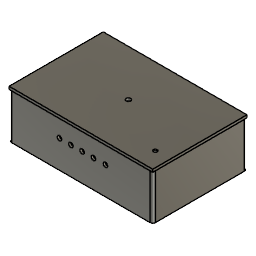
Modelado 3D rehechov2 (Autodesk Fusion 360 design; units mm, degrees)
part number: 2026-04-29-23-24-20-997
part number: 2026-04-29-23-24-29-026
Autodesk Fusion 360 part; units mm, degrees
sketch "Boceto1" plane through (0, 0, 0) normal (0, 0, 1) x (1, 0, 0) in component "PrototipoUV_CajaReal"
  line L0 (0, 0) -> (160, 0)
  line L1 (160, 0) -> (160, 105)
  line L2 (160, 105) -> (0, 105)
  line L3 (0, 105) -> (0, 0)
extrude "Extruir1" add sketch "Boceto1" along normal blind 50 makes body 1 in component "PrototipoUV_CajaReal"
fillet "Empalme1" radius 3 4 edges at (0, 105, 25) (160, 105, 25) (160, 0, 25) (0, 0, 25) on bodies 1 in component "PrototipoUV_CajaReal"
shell "Vaciado1" thickness 2.5 removed faces 1 at (105.6667, 35, 50) on bodies 1 in component "PrototipoUV_CajaReal"
ref_plane "PlanoDeObra1" through (0, 0, 50) normal (0, 0, 1) x (1, 0, 0) in component "PrototipoUV_CajaReal"
sketch "Boceto2" plane through (0, 0, 50) normal (0, 0, 1) x (1, 0, 0) in component "PrototipoUV_CajaReal"
  line L0 (0, 0) -> (160, 0)
  line L1 (160, 0) -> (160, 105)
  line L2 (160, 105) -> (0, 105)
  line L3 (0, 105) -> (0, 0)
extrude "Extruir2" add sketch "Boceto2" along normal blind 3 separate body makes body 2 in component "PrototipoUV_CajaReal"
ref_plane "PlanoDeObra2" through (0, 0, 46.5) normal (0, 0, 1) x (1, 0, 0) in component "PrototipoUV_CajaReal"
sketch "Boceto3" plane through (0, 0, 46.5) normal (0, 0, 1) x (1, 0, 0) in component "PrototipoUV_CajaReal"
  line L0 (3.7, 3.7) -> (156.3, 3.7)
  line L1 (156.3, 3.7) -> (156.3, 101.3)
  line L2 (156.3, 101.3) -> (3.7, 101.3)
  line L3 (3.7, 101.3) -> (3.7, 3.7)
extrude "Extruir3" add sketch "Boceto3" along normal blind 3.5 separate body makes body 3 in component "PrototipoUV_CajaReal"
ref_plane "PlanoDeObra3" through (0, 0, 53.3) normal (0, 0, 1) x (1, 0, 0) in component "PrototipoUV_CajaReal"
sketch "Boceto4" plane through (0, 0, 53.3) normal (0, 0, 1) x (1, 0, 0) in component "PrototipoUV_CajaReal"
  line L0 (30, 12.5) -> (130, 12.5)
  line L1 (130, 12.5) -> (130, 92.5)
  line L2 (130, 92.5) -> (30, 92.5)
  line L3 (30, 92.5) -> (30, 12.5)
ref_plane "PlanoDeObra4" through (0, 0, 55.2) normal (0, 0, 1) x (1, 0, 0) in component "PrototipoUV_CajaReal"
sketch "Boceto5" plane through (0, 0, 55.2) normal (0, 0, 1) x (1, 0, 0) in component "PrototipoUV_CajaReal"
  line L0 (30, 12.5) -> (130, 12.5)
  line L1 (130, 12.5) -> (130, 13.7)
  line L2 (130, 13.7) -> (30, 13.7)
  line L3 (30, 13.7) -> (30, 12.5)
ref_plane "PlanoDeObra5" through (0, 0, 55.2) normal (0, 0, 1) x (1, 0, 0) in component "PrototipoUV_CajaReal"
sketch "Boceto6" plane through (0, 0, 55.2) normal (0, 0, 1) x (1, 0, 0) in component "PrototipoUV_CajaReal"
  line L0 (30, 91.3) -> (130, 91.3)
  line L1 (130, 91.3) -> (130, 92.5)
  line L2 (130, 92.5) -> (30, 92.5)
  line L3 (30, 92.5) -> (30, 91.3)
ref_plane "PlanoDeObra6" through (0, 0, 55.2) normal (0, 0, 1) x (1, 0, 0) in component "PrototipoUV_CajaReal"
sketch "Boceto7" plane through (0, 0, 55.2) normal (0, 0, 1) x (1, 0, 0) in component "PrototipoUV_CajaReal"
  line L0 (30, 12.5) -> (31.2, 12.5)
  line L1 (31.2, 12.5) -> (31.2, 92.5)
  line L2 (31.2, 92.5) -> (30, 92.5)
  line L3 (30, 92.5) -> (30, 12.5)
ref_plane "PlanoDeObra7" through (0, 0, 55.2) normal (0, 0, 1) x (1, 0, 0) in component "PrototipoUV_CajaReal"
sketch "Boceto8" plane through (0, 0, 55.2) normal (0, 0, 1) x (1, 0, 0) in component "PrototipoUV_CajaReal"
  line L0 (128.8, 12.5) -> (130, 12.5)
  line L1 (130, 12.5) -> (130, 92.5)
  line L2 (130, 92.5) -> (128.8, 92.5)
  line L3 (128.8, 92.5) -> (128.8, 12.5)
ref_plane "PlanoDeObra8" through (0, 0, 55.25) normal (0, 0, 1) x (1, 0, 0) in component "PrototipoUV_CajaReal"
sketch "Boceto9" plane through (0, 0, 55.25) normal (0, 0, 1) x (1, 0, 0) in component "PrototipoUV_CajaReal"
  line L0 (54.75, 14) -> (55.25, 14)
  line L1 (55.25, 14) -> (55.25, 91)
  line L2 (55.25, 91) -> (54.75, 91)
  line L3 (54.75, 91) -> (54.75, 14)
ref_plane "PlanoDeObra9" through (0, 0, 55.25) normal (0, 0, 1) x (1, 0, 0) in component "PrototipoUV_CajaReal"
sketch "Boceto10" plane through (0, 0, 55.25) normal (0, 0, 1) x (1, 0, 0) in component "PrototipoUV_CajaReal"
  line L0 (79.75, 14) -> (80.25, 14)
  line L1 (80.25, 14) -> (80.25, 91)
  line L2 (80.25, 91) -> (79.75, 91)
  line L3 (79.75, 91) -> (79.75, 14)
ref_plane "PlanoDeObra10" through (0, 0, 55.25) normal (0, 0, 1) x (1, 0, 0) in component "PrototipoUV_CajaReal"
sketch "Boceto11" plane through (0, 0, 55.25) normal (0, 0, 1) x (1, 0, 0) in component "PrototipoUV_CajaReal"
  line L0 (104.75, 14) -> (105.25, 14)
  line L1 (105.25, 14) -> (105.25, 91)
  line L2 (105.25, 91) -> (104.75, 91)
  line L3 (104.75, 91) -> (104.75, 14)
ref_plane "PlanoDeObra11" through (0, 0, 55.25) normal (0, 0, 1) x (1, 0, 0) in component "PrototipoUV_CajaReal"
sketch "Boceto12" plane through (0, 0, 55.25) normal (0, 0, 1) x (1, 0, 0) in component "PrototipoUV_CajaReal"
  line L0 (31.5, 38.9167) -> (128.5, 38.9167)
  line L1 (128.5, 38.9167) -> (128.5, 39.4167)
  line L2 (128.5, 39.4167) -> (31.5, 39.4167)
  line L3 (31.5, 39.4167) -> (31.5, 38.9167)
ref_plane "PlanoDeObra12" through (0, 0, 55.25) normal (0, 0, 1) x (1, 0, 0) in component "PrototipoUV_CajaReal"
sketch "Boceto13" plane through (0, 0, 55.25) normal (0, 0, 1) x (1, 0, 0) in component "PrototipoUV_CajaReal"
  line L0 (31.5, 65.5833) -> (128.5, 65.5833)
  line L1 (128.5, 65.5833) -> (128.5, 66.0833)
  line L2 (128.5, 66.0833) -> (31.5, 66.0833)
  line L3 (31.5, 66.0833) -> (31.5, 65.5833)
ref_plane "PlanoDeObra13" through (0, 0, 53.3) normal (0, 0, 1) x (1, 0, 0) in component "PrototipoUV_CajaReal"
sketch "Boceto14" plane through (0, 0, 53.3) normal (0, 0, 1) x (1, 0, 0) in component "PrototipoUV_CajaReal"
  line L0 (134.5, 17.5) -> (151.5, 17.5)
  line L1 (151.5, 17.5) -> (151.5, 32.5)
  line L2 (151.5, 32.5) -> (134.5, 32.5)
  line L3 (134.5, 32.5) -> (134.5, 17.5)
ref_plane "PlanoDeObra14" through (0, 0, 54.6) normal (0, 0, 1) x (1, 0, 0) in component "PrototipoUV_CajaReal"
sketch "Boceto15" plane through (0, 0, 54.6) normal (0, 0, 1) x (1, 0, 0) in component "PrototipoUV_CajaReal"
  circle A0 centre (143, 25) radius 2.8
ref_plane "PlanoDeObra15" through (0, -0.6, 0) normal (0, 1, 0) x (0, 0, 1) in component "PrototipoUV_CajaReal"
sketch "Boceto16" plane through (0, -0.6, 0) normal (0, 1, 0) x (1, 0, 0) in component "PrototipoUV_CajaReal"
  circle A0 centre (80, 23.5) radius 4
ref_plane "PlanoDeObra16" through (0, 105.1, 0) normal (0, 1, 0) x (0, 0, 1) in component "PrototipoUV_CajaReal"
sketch "Boceto17" plane through (0, 105.1, 0) normal (0, 1, 0) x (1, 0, 0) in component "PrototipoUV_CajaReal"
  circle A0 centre (108, 16) radius 1.25
ref_plane "PlanoDeObra17" through (0, 105.1, 0) normal (0, 1, 0) x (0, 0, 1) in component "PrototipoUV_CajaReal"
sketch "Boceto18" plane through (0, 105.1, 0) normal (0, 1, 0) x (1, 0, 0) in component "PrototipoUV_CajaReal"
  circle A0 centre (113.5, 16) radius 1.25
ref_plane "PlanoDeObra18" through (0, 105.1, 0) normal (0, 1, 0) x (0, 0, 1) in component "PrototipoUV_CajaReal"
sketch "Boceto19" plane through (0, 105.1, 0) normal (0, 1, 0) x (1, 0, 0) in component "PrototipoUV_CajaReal"
  circle A0 centre (119, 16) radius 1.25
ref_plane "PlanoDeObra19" through (0, 105.1, 0) normal (0, 1, 0) x (0, 0, 1) in component "PrototipoUV_CajaReal"
sketch "Boceto20" plane through (0, 105.1, 0) normal (0, 1, 0) x (1, 0, 0) in component "PrototipoUV_CajaReal"
  circle A0 centre (124.5, 16) radius 1.25
ref_plane "PlanoDeObra20" through (0, 105.1, 0) normal (0, 1, 0) x (0, 0, 1) in component "PrototipoUV_CajaReal"
sketch "Boceto21" plane through (0, 105.1, 0) normal (0, 1, 0) x (1, 0, 0) in component "PrototipoUV_CajaReal"
  circle A0 centre (130, 16) radius 1.25
ref_plane "PlanoDeObra21" through (0, 105.1, 0) normal (0, 1, 0) x (0, 0, 1) in component "PrototipoUV_CajaReal"
sketch "Boceto22" plane through (0, 105.1, 0) normal (0, 1, 0) x (1, 0, 0) in component "PrototipoUV_CajaReal"
  circle A0 centre (135.5, 16) radius 1.25
ref_plane "PlanoDeObra22" through (0, 105.1, 0) normal (0, 1, 0) x (0, 0, 1) in component "PrototipoUV_CajaReal"
sketch "Boceto23" plane through (0, 105.1, 0) normal (0, 1, 0) x (1, 0, 0) in component "PrototipoUV_CajaReal"
  circle A0 centre (141, 16) radius 1.25
ref_plane "PlanoDeObra23" through (0, 105.1, 0) normal (0, 1, 0) x (0, 0, 1) in component "PrototipoUV_CajaReal"
sketch "Boceto24" plane through (0, 105.1, 0) normal (0, 1, 0) x (1, 0, 0) in component "PrototipoUV_CajaReal"
  circle A0 centre (146.5, 16) radius 1.25
ref_plane "PlanoDeObra24" through (0, 105.1, 0) normal (0, 1, 0) x (0, 0, 1) in component "PrototipoUV_CajaReal"
sketch "Boceto25" plane through (0, 105.1, 0) normal (0, 1, 0) x (1, 0, 0) in component "PrototipoUV_CajaReal"
  circle A0 centre (108, 21.5) radius 1.25
ref_plane "PlanoDeObra25" through (0, 105.1, 0) normal (0, 1, 0) x (0, 0, 1) in component "PrototipoUV_CajaReal"
sketch "Boceto26" plane through (0, 105.1, 0) normal (0, 1, 0) x (1, 0, 0) in component "PrototipoUV_CajaReal"
  circle A0 centre (113.5, 21.5) radius 1.25
ref_plane "PlanoDeObra26" through (0, 105.1, 0) normal (0, 1, 0) x (0, 0, 1) in component "PrototipoUV_CajaReal"
sketch "Boceto27" plane through (0, 105.1, 0) normal (0, 1, 0) x (1, 0, 0) in component "PrototipoUV_CajaReal"
  circle A0 centre (119, 21.5) radius 1.25
ref_plane "PlanoDeObra27" through (0, 105.1, 0) normal (0, 1, 0) x (0, 0, 1) in component "PrototipoUV_CajaReal"
sketch "Boceto28" plane through (0, 105.1, 0) normal (0, 1, 0) x (1, 0, 0) in component "PrototipoUV_CajaReal"
  circle A0 centre (124.5, 21.5) radius 1.25
ref_plane "PlanoDeObra28" through (0, 105.1, 0) normal (0, 1, 0) x (0, 0, 1) in component "PrototipoUV_CajaReal"
sketch "Boceto29" plane through (0, 105.1, 0) normal (0, 1, 0) x (1, 0, 0) in component "PrototipoUV_CajaReal"
  circle A0 centre (130, 21.5) radius 1.25
ref_plane "PlanoDeObra29" through (0, 105.1, 0) normal (0, 1, 0) x (0, 0, 1) in component "PrototipoUV_CajaReal"
sketch "Boceto30" plane through (0, 105.1, 0) normal (0, 1, 0) x (1, 0, 0) in component "PrototipoUV_CajaReal"
  circle A0 centre (135.5, 21.5) radius 1.25
ref_plane "PlanoDeObra30" through (0, 105.1, 0) normal (0, 1, 0) x (0, 0, 1) in component "PrototipoUV_CajaReal"
sketch "Boceto31" plane through (0, 105.1, 0) normal (0, 1, 0) x (1, 0, 0) in component "PrototipoUV_CajaReal"
  circle A0 centre (141, 21.5) radius 1.25
ref_plane "PlanoDeObra31" through (0, 105.1, 0) normal (0, 1, 0) x (0, 0, 1) in component "PrototipoUV_CajaReal"
sketch "Boceto32" plane through (0, 105.1, 0) normal (0, 1, 0) x (1, 0, 0) in component "PrototipoUV_CajaReal"
  circle A0 centre (146.5, 21.5) radius 1.25
ref_plane "PlanoDeObra32" through (0, 105.1, 0) normal (0, 1, 0) x (0, 0, 1) in component "PrototipoUV_CajaReal"
sketch "Boceto33" plane through (0, 105.1, 0) normal (0, 1, 0) x (1, 0, 0) in component "PrototipoUV_CajaReal"
  circle A0 centre (108, 27) radius 1.25
ref_plane "PlanoDeObra33" through (0, 105.1, 0) normal (0, 1, 0) x (0, 0, 1) in component "PrototipoUV_CajaReal"
sketch "Boceto34" plane through (0, 105.1, 0) normal (0, 1, 0) x (1, 0, 0) in component "PrototipoUV_CajaReal"
  circle A0 centre (113.5, 27) radius 1.25
ref_plane "PlanoDeObra34" through (0, 105.1, 0) normal (0, 1, 0) x (0, 0, 1) in component "PrototipoUV_CajaReal"
sketch "Boceto35" plane through (0, 105.1, 0) normal (0, 1, 0) x (1, 0, 0) in component "PrototipoUV_CajaReal"
  circle A0 centre (119, 27) radius 1.25
ref_plane "PlanoDeObra35" through (0, 105.1, 0) normal (0, 1, 0) x (0, 0, 1) in component "PrototipoUV_CajaReal"
sketch "Boceto36" plane through (0, 105.1, 0) normal (0, 1, 0) x (1, 0, 0) in component "PrototipoUV_CajaReal"
  circle A0 centre (124.5, 27) radius 1.25
ref_plane "PlanoDeObra36" through (0, 105.1, 0) normal (0, 1, 0) x (0, 0, 1) in component "PrototipoUV_CajaReal"
sketch "Boceto37" plane through (0, 105.1, 0) normal (0, 1, 0) x (1, 0, 0) in component "PrototipoUV_CajaReal"
  circle A0 centre (130, 27) radius 1.25
ref_plane "PlanoDeObra37" through (0, 105.1, 0) normal (0, 1, 0) x (0, 0, 1) in component "PrototipoUV_CajaReal"
sketch "Boceto38" plane through (0, 105.1, 0) normal (0, 1, 0) x (1, 0, 0) in component "PrototipoUV_CajaReal"
  circle A0 centre (135.5, 27) radius 1.25
ref_plane "PlanoDeObra38" through (0, 105.1, 0) normal (0, 1, 0) x (0, 0, 1) in component "PrototipoUV_CajaReal"
sketch "Boceto39" plane through (0, 105.1, 0) normal (0, 1, 0) x (1, 0, 0) in component "PrototipoUV_CajaReal"
  circle A0 centre (141, 27) radius 1.25
ref_plane "PlanoDeObra39" through (0, 105.1, 0) normal (0, 1, 0) x (0, 0, 1) in component "PrototipoUV_CajaReal"
sketch "Boceto40" plane through (0, 105.1, 0) normal (0, 1, 0) x (1, 0, 0) in component "PrototipoUV_CajaReal"
  circle A0 centre (146.5, 27) radius 1.25
ref_plane "PlanoDeObra40" through (0, 0, 3) normal (0, 0, 1) x (1, 0, 0) in component "PrototipoUV_CajaReal"
sketch "Boceto41" plane through (0, 0, 3) normal (0, 0, 1) x (1, 0, 0) in component "PrototipoUV_CajaReal"
  line L0 (12.5, 12.5) -> (75.5, 12.5)
  line L1 (75.5, 12.5) -> (75.5, 39.5)
  line L2 (75.5, 39.5) -> (12.5, 39.5)
  line L3 (12.5, 39.5) -> (12.5, 12.5)
ref_plane "PlanoDeObra41" through (0, 0, 3) normal (0, 0, 1) x (1, 0, 0) in component "PrototipoUV_CajaReal"
sketch "Boceto42" plane through (0, 0, 3) normal (0, 0, 1) x (1, 0, 0) in component "PrototipoUV_CajaReal"
  line L0 (94, 12.5) -> (149, 12.5)
  line L1 (149, 12.5) -> (149, 47.5)
  line L2 (149, 47.5) -> (94, 47.5)
  line L3 (94, 47.5) -> (94, 12.5)
sketch "Boceto1 (2)" plane through (0, 0, 0) normal (0, -1, 0) x (1, 0, 0)
  line L0 (3, 50) -> (3, 0)
  line L1 (3, 0) -> (157, 0)
  line L2 (157, 0) -> (157, 50)
  line L3 (157, 50) -> (3, 50)
hole "Agujero1" at (80, 105, 25) direction (0, -1, 0) diameter 8 depth 5 tip angle 118 bodies 1 in component "PrototipoUV_CajaReal"
sketch "Boceto2 (2)" plane through (0, 0, 0) normal (0, 1, 0) x (1, 0, 0)
sketch "Boceto3 (2)" plane through (0, 0, 0) normal (0, 1, 0) x (1, 0, 0)
sketch "Boceto4 (2)" plane through (0, 0, 0) normal (0, 1, 0) x (1, 0, 0)
  circle A0 centre (40, -30) radius 2.5
  circle A1 centre (40, -30) radius 2.5
  circle A2 centre (50, -30) radius 2.5
  circle A3 centre (60, -30) radius 2.5
  circle A4 centre (70, -30) radius 2.5
  circle A5 centre (80, -30) radius 2.5
  circle A6 centre (90, -30) radius 2.5
  circle A7 centre (100, -30) radius 2.5
  dimension "d132" = 5
  dimension "d133" = 5
  dimension "d134" = 5
  dimension "d135" = 5
  dimension "d136" = 5
  dimension "d137" = 5
  dimension "d138" = 5
  dimension "d139" = 5
  measures "d132" diameter of A0
  measures "d133" diameter of A1
  measures "d134" diameter of A2
  measures "d135" diameter of A3
  measures "d136" diameter of A4
  measures "d137" diameter of A5
  measures "d138" diameter of A6
  measures "d139" diameter of A7
hole "Agujero9" at (107.3794, 2.5, 30.9159) direction (0, -1, 0) diameter 5 depth 30 tip angle 118 bodies 1 in component "PrototipoUV_CajaReal"
hole "Agujero10" at (94.084, 2.5, 30.8935) direction (0, -1, 0) diameter 5 depth 30 tip angle 118 bodies 1 in component "PrototipoUV_CajaReal"
hole "Agujero11" at (81.3834, 2.5, 30.8721) direction (0, -1, 0) diameter 5 depth 30 tip angle 118 bodies 1 in component "PrototipoUV_CajaReal"
hole "Agujero12" at (68.9096, 2.5, 30.8512) direction (0, -1, 0) diameter 5 depth 30 tip angle 118 bodies 1 in component "PrototipoUV_CajaReal"
hole "Agujero13" at (56.209, 2.5, 31.0624) direction (0, -1, 0) diameter 5 depth 30 tip angle 118 bodies 1 in component "PrototipoUV_CajaReal"
sketch "Boceto9 (2)" plane through (0, 0, 2.5) normal (0, 0, 1) x (-1, 0, 0)
  arc A0 (-2.5, -3) -> (-3, -2.5) centre (-3, -3) ccw
  line L0 (-3, -2.5) -> (-157, -2.5)
  arc A1 (-157, -2.5) -> (-157.5, -3) centre (-157, -3) ccw
  line L1 (-157.5, -3) -> (-157.5, -102)
  arc A2 (-157.5, -102) -> (-157, -102.5) centre (-157, -102) ccw
  line L2 (-157, -102.5) -> (-3, -102.5)
  arc A3 (-3, -102.5) -> (-2.5, -102) centre (-3, -102) ccw
  line L3 (-2.5, -102) -> (-2.5, -3)
  line L4 (-150, -10) -> (-94, -10)
  line L5 (-94, -10) -> (-94, -13)
  line L6 (-94, -13) -> (-150, -13)
  line L7 (-150, -13) -> (-150, -10)
  line L8 (-147.3696, -10) -> (-150.3696, -10)
  line L9 (-150.3696, -10) -> (-150.3696, -45)
  line L10 (-150.3696, -45) -> (-147.3696, -45)
  line L11 (-147.3696, -45) -> (-147.3696, -10)
  line L12 (-150.3696, -41.6297) -> (-94.3696, -41.6297)
  line L13 (-94.3696, -41.6297) -> (-94.3696, -45)
  line L14 (-94.3696, -45) -> (-150.3696, -45)
  line L15 (-150.3696, -45) -> (-150.3696, -41.6297)
  dimension "d190" = 56
  dimension "d191" = 3
  dimension "d192" = 3
  dimension "d193" = 35
  dimension "d194" = 56
  constraint horizontal L4
  constraint vertical L5
  constraint horizontal L6
  constraint vertical L7
  constraint horizontal L8
  constraint vertical L9
  constraint horizontal L10
  constraint vertical L11
  constraint coincident L4 L8.start
  constraint horizontal L12
  constraint vertical L13
  constraint horizontal L14
  constraint vertical L15
  constraint coincident L9 L12.start
  measures "d190" distance of L4.start L4.end
  measures "d191" distance of L4.start L6.end
  measures "d192" distance of L8.start L8.end
  measures "d193" distance of L8.start L10.end
  measures "d194" distance of L12.start L12.end
extrude "Extruir46" add sketch "Boceto9 (2)" along normal blind 10 contours L4 L6 L7 L8 L11 | L6 L7 L8 L9 L11 L12 | L4 L5 L6 L11 | L9 L10 L11 L12 L14 L15 | L11 L12 L13 L14 bodies 1 in component "PrototipoUV_CajaReal"
sketch "Boceto10 (2)" plane through (0, 0, 4.5) normal (0, 0, 1) x (-1, 0, 0)
  line L0 (-12.5, -39.5) -> (-12.5, -12.5)
  line L1 (-12.5, -12.5) -> (-75.5, -12.5)
  line L2 (-75.5, -12.5) -> (-75.5, -39.5)
  line L3 (-75.5, -39.5) -> (-12.5, -39.5)
  line L4 (-150, -52.9904) -> (-82, -52.9904)
  line L5 (-82, -52.9904) -> (-82, -49.9904)
  line L6 (-82, -49.9904) -> (-150, -49.9904)
  line L7 (-150, -49.9904) -> (-150, -52.9904)
  line L8 (-150, -49.9904) -> (-147, -49.9904)
  line L9 (-147, -49.9904) -> (-147, -100.9904)
  line L10 (-147, -100.9904) -> (-150, -100.9904)
  line L11 (-150, -100.9904) -> (-150, -49.9904)
  line L12 (-150, -100.9904) -> (-82, -100.9904)
  line L13 (-82, -100.9904) -> (-82, -97.9904)
  line L14 (-82, -97.9904) -> (-150, -97.9904)
  line L15 (-150, -97.9904) -> (-150, -100.9904)
  dimension "d197" = 68
  dimension "d198" = 3
  dimension "d199" = 3
  dimension "d200" = 51
  dimension "d201" = 68
  dimension "d202" = 3
  constraint horizontal L4
  constraint vertical L5
  constraint horizontal L6
  constraint vertical L7
  constraint horizontal L8
  constraint vertical L9
  constraint horizontal L10
  constraint vertical L11
  constraint horizontal L12
  constraint vertical L13
  constraint horizontal L14
  constraint vertical L15
  measures "d197" distance of L4.start L4.end
  measures "d198" distance of L4.start L6.end
  measures "d199" distance of L6.end L8.end
  measures "d200" distance of L6.end L10.end
  measures "d201" distance of L10.end L12.end
  measures "d202" distance of L10.end L14.end
extrude "Extruir1'" add sketch "Boceto10 (2)" along normal blind 9 separate body contours L4 L6 L7 L8 L9 L11 | L4 L9 L11 L14 | L4 L5 L6 L9 | L9 L10 L11 L12 L14 L15 | L9 L12 L13 L14 makes body 4
hole "Agujero14" at (143.6047, 19.3786, 53) direction (0, 0, -1) diameter 3.3 depth 7 tip angle 180 countersink diameter 4.4 countersink angle 90 bodies 2 3 in component "PrototipoUV_CajaReal"
hole "Agujero17" at (79.3666, 53.5561, 53) direction (0, 0, -1) diameter 5 depth 7 tip angle 180 bodies 2 3 in component "PrototipoUV_CajaReal"
sketch "Boceto11 (2)" plane through (0, 0, 2.5) normal (0, 0, 1) x (-1, 0, 0)
  line L0 (-147.3696, -41.6297) -> (-94.3696, -41.6297)
  line L1 (-94.3696, -41.6297) -> (-94.3696, -45)
  line L2 (-94.3696, -45) -> (-150.3696, -45)
  line L3 (-150.3696, -45) -> (-150.3696, -10)
  line L4 (-150.3696, -10) -> (-94, -10)
  line L5 (-94, -10) -> (-94, -13)
  line L6 (-94, -13) -> (-147.3696, -13)
  line L7 (-147.3696, -13) -> (-147.3696, -41.6297)
  arc A0 (-2.5, -3) -> (-3, -2.5) centre (-3, -3) ccw
  line L8 (-3, -2.5) -> (-157, -2.5)
  arc A1 (-157, -2.5) -> (-157.5, -3) centre (-157, -3) ccw
  line L9 (-157.5, -3) -> (-157.5, -102)
  arc A2 (-157.5, -102) -> (-157, -102.5) centre (-157, -102) ccw
  line L10 (-157, -102.5) -> (-3, -102.5)
  arc A3 (-3, -102.5) -> (-2.5, -102) centre (-3, -102) ccw
  line L11 (-2.5, -102) -> (-2.5, -3)
  line L12 (-9.5188, -94.9305) -> (-57.5188, -94.9305)
  line L13 (-57.5188, -94.9305) -> (-57.5188, -91.9305)
  line L14 (-57.5188, -91.9305) -> (-9.5188, -91.9305)
  line L15 (-9.5188, -91.9305) -> (-9.5188, -94.9305)
  line L16 (-9.5188, -94.9305) -> (-12.5188, -94.9305)
  line L17 (-12.5188, -94.9305) -> (-12.5188, -59.9305)
  line L18 (-12.5188, -59.9305) -> (-9.5188, -59.9305)
  line L19 (-9.5188, -59.9305) -> (-9.5188, -94.9305)
  line L20 (-9.5188, -59.9305) -> (-57.5188, -59.9305)
  line L21 (-57.5188, -59.9305) -> (-57.5188, -62.9305)
  line L22 (-57.5188, -62.9305) -> (-9.5188, -62.9305)
  line L23 (-9.5188, -62.9305) -> (-9.5188, -59.9305)
  dimension "d223" = 48
  dimension "d224" = 3
  dimension "d225" = 3
  dimension "d226" = 35
  dimension "d227" = 48
  dimension "d228" = 3
  constraint horizontal L12
  constraint vertical L13
  constraint horizontal L14
  constraint vertical L15
  constraint horizontal L16
  constraint vertical L17
  constraint horizontal L18
  constraint vertical L19
  constraint horizontal L20
  constraint vertical L21
  constraint horizontal L22
  constraint vertical L23
  measures "d223" distance of L12.start L12.end
  measures "d224" distance of L12.start L14.end
  measures "d225" distance of L12.start L16.end
  measures "d226" distance of L12.start L18.end
  measures "d227" distance of L18.end L20.end
  measures "d228" distance of L18.end L22.end
extrude "Extruir47" add sketch "Boceto11 (2)" along normal blind 9 contours L12 L14 L15 L16 L17 L19 | L12 L13 L14 L17 | L14 L17 L19 L22 | L17 L18 L19 L20 L22 L23 | L17 L20 L21 L22 bodies 1 in component "PrototipoUV_CajaReal"
hole "Agujero18" at (76.0734, 18.3409, 2.5) direction (0, 0, -1) diameter 5.05 depth 3 tip angle 118 bodies 1 in component "PrototipoUV_CajaReal"
hole "Agujero19" at (66.6169, 29.1493, 2.5) direction (0, 0, -1) diameter 5.05 depth 3 tip angle 118 bodies 1 in component "PrototipoUV_CajaReal"
hole "Agujero2" [suppressed] in component "PrototipoUV_CajaReal"
hole "Agujero3" [suppressed] in component "PrototipoUV_CajaReal"
hole "Agujero4" [suppressed] in component "PrototipoUV_CajaReal"
hole "Agujero5" [suppressed] in component "PrototipoUV_CajaReal"
hole "Agujero6" [suppressed] in component "PrototipoUV_CajaReal"
hole "Agujero7" [suppressed] in component "PrototipoUV_CajaReal"
hole "Agujero8" [suppressed] in component "PrototipoUV_CajaReal"
sketch "Boceto7 (2)" plane through (0, 0, 2.5) normal (0, 0, 1) x (-1, 0, 0)
  arc A0 (-2.5, -3) -> (-3, -2.5) centre (-3, -3) ccw
  line L0 (-3, -2.5) -> (-157, -2.5)
  arc A1 (-157, -2.5) -> (-157.5, -3) centre (-157, -3) ccw
  line L1 (-157.5, -3) -> (-157.5, -102)
  arc A2 (-157.5, -102) -> (-157, -102.5) centre (-157, -102) ccw
  line L2 (-157, -102.5) -> (-3, -102.5)
  arc A3 (-3, -102.5) -> (-2.5, -102) centre (-3, -102) ccw
  line L3 (-2.5, -102) -> (-2.5, -3)
  line L4 (-150, -10) -> (-94, -10)
  line L5 (-94, -10) -> (-94, -13)
  line L6 (-94, -13) -> (-150, -13)
  line L7 (-150, -13) -> (-150, -10)
  line L8 (-150, -10) -> (-147, -10)
  line L9 (-147, -10) -> (-147, -45)
  line L10 (-147, -45) -> (-150, -45)
  line L11 (-150, -45) -> (-150, -10)
  line L12 (-150, -45) -> (-94, -45)
  line L13 (-94, -45) -> (-94, -48)
  line L14 (-94, -48) -> (-150, -48)
  line L15 (-150, -48) -> (-150, -45)
  dimension "d167" = 56
  dimension "d168" = 3
  dimension "d169" = 3
  dimension "d170" = 35
  dimension "d171" = 56
  dimension "d172" = 3
  constraint horizontal L4
  constraint vertical L5
  constraint horizontal L6
  constraint vertical L7
  constraint horizontal L8
  constraint vertical L9
  constraint horizontal L10
  constraint vertical L11
  constraint horizontal L12
  constraint vertical L13
  constraint horizontal L14
  constraint vertical L15
  measures "d167" distance of L4.start L4.end
  measures "d168" distance of L4.start L6.end
  measures "d169" distance of L4.start L8.end
  measures "d170" distance of L4.start L10.end
  measures "d171" distance of L10.end L12.end
  measures "d172" distance of L10.end L14.end
extrude "Extruir45" [suppressed] in component "PrototipoUV_CajaReal"
move_body "Desplazar1" [suppressed] in component "PrototipoUV_CajaReal"
move_body "Desplazar2" [suppressed] in component "PrototipoUV_CajaReal"
move_body "Desplazar3" [suppressed] in component "PrototipoUV_CajaReal"
sketch "Boceto8 (2)" plane through (0, 0, -0.0582) normal (0, 0, 1) x (-1, 0, 0)
  line L0 (-155.3931, -44.8161) -> (-155.3931, -6.8161)
  line L1 (-155.3931, -6.8161) -> (-99.3931, -6.8161)
  line L2 (-99.3931, -6.8161) -> (-99.3931, -9.8161)
  line L3 (-99.3931, -9.8161) -> (-152.3931, -9.8161)
  line L4 (-152.3931, -9.8161) -> (-152.3931, -41.8161)
  line L5 (-152.3931, -41.8161) -> (-99.3931, -41.8161)
  line L6 (-99.3931, -41.8161) -> (-99.3931, -44.8161)
  line L7 (-99.3931, -44.8161) -> (-155.3931, -44.8161)
  arc A0 (-7.8931, 0.1839) -> (-8.3931, 0.6839) centre (-8.3931, 0.1839) ccw
  line L8 (-8.3931, 0.6839) -> (-162.3931, 0.6839)
  arc A1 (-162.3931, 0.6839) -> (-162.8931, 0.1839) centre (-162.3931, 0.1839) ccw
  line L9 (-162.8931, 0.1839) -> (-162.8931, -98.8161)
  arc A2 (-162.8931, -98.8161) -> (-162.3931, -99.3161) centre (-162.3931, -98.8161) ccw
  line L10 (-162.3931, -99.3161) -> (-8.3931, -99.3161)
  arc A3 (-8.3931, -99.3161) -> (-7.8931, -98.8161) centre (-8.3931, -98.8161) ccw
  line L11 (-7.8931, -98.8161) -> (-7.8931, 0.1839)
sketch "Boceto5 (2)" plane through (0, 0, 2.5) normal (0, 0, 1) x (-1, 0, 0)
  arc A0 (-2.5, -3) -> (-3, -2.5) centre (-3, -3) ccw
  line L0 (-3, -2.5) -> (-157, -2.5)
  arc A1 (-157, -2.5) -> (-157.5, -3) centre (-157, -3) ccw
  line L1 (-157.5, -3) -> (-157.5, -102)
  arc A2 (-157.5, -102) -> (-157, -102.5) centre (-157, -102) ccw
  line L2 (-157, -102.5) -> (-3, -102.5)
  arc A3 (-3, -102.5) -> (-2.5, -102) centre (-3, -102) ccw
  line L3 (-2.5, -102) -> (-2.5, -3)
  line L4 (-150, -15) -> (-93.6658, -15)
  line L5 (-93.6658, -15) -> (-93.6658, -14.8495)
  line L6 (-93.6658, -14.8495) -> (-150, -14.8495)
  line L7 (-150, -14.8495) -> (-150, -15)
  line L8 (-93.6658, -15) -> (-153.4444, -15)
  line L9 (-153.4444, -15) -> (-153.4444, -51.0212)
  line L10 (-153.4444, -51.0212) -> (-93.6658, -51.0212)
  line L11 (-93.6658, -51.0212) -> (-93.6658, -15)
  line L12 (-154.9414, -12.8858) -> (-91.48, -12.8858)
  line L13 (-91.48, -12.8858) -> (-91.48, -12.6382)
  line L14 (-91.48, -12.6382) -> (-154.9414, -12.6382)
  line L15 (-154.9414, -12.6382) -> (-154.9414, -12.8858)
  line L16 (-91.48, -53.3942) -> (-154.9414, -53.3942)
  line L17 (-154.9414, -53.3942) -> (-154.9414, -52.6314)
  line L18 (-154.9414, -52.6314) -> (-91.48, -52.6314)
  line L19 (-91.48, -52.6314) -> (-91.48, -53.3942)
  line L20 (-154.9414, -12.8858) -> (-91.48, -12.8858)
  line L21 (-91.48, -12.8858) -> (-91.48, -52.6314)
  line L22 (-91.48, -52.6314) -> (-154.9414, -52.6314)
  line L23 (-154.9414, -52.6314) -> (-154.9414, -12.8858)
  constraint horizontal L4
  constraint vertical L5
  constraint horizontal L6
  constraint vertical L7
  constraint horizontal L8
  constraint vertical L9
  constraint horizontal L10
  constraint vertical L11
  constraint horizontal L12
  constraint vertical L13
  constraint horizontal L14
  constraint vertical L15
  constraint horizontal L16
  constraint vertical L17
  constraint horizontal L18
  constraint vertical L19
  constraint horizontal L20
  constraint vertical L21
  constraint horizontal L22
  constraint vertical L23
extrude "Extruir43" [suppressed] in component "PrototipoUV_CajaReal"
sketch "Boceto6 (2)" plane through (0, 0, 4.5) normal (0, 0, 1) x (-1, 0, 0)
  line L0 (-12.5, -39.5) -> (-12.5, -12.5)
  line L1 (-12.5, -12.5) -> (-75.5, -12.5)
  line L2 (-75.5, -12.5) -> (-75.5, -39.5)
  line L3 (-75.5, -39.5) -> (-12.5, -39.5)
extrude "Extruir44" [suppressed] in component "PrototipoUV_CajaReal"
component "PrototipoUV_CajaReal" placed x (1, 0, 0) y (0, 1, 0) z (0, 0, 1) at (0, 0, 0)
named bodies: "Carcasa_Base_abierta", "Tapa_superior_cerrada", "Labio_interior_tapa"
